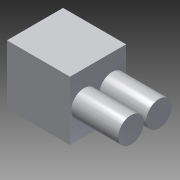
# Autodesk Inventor part: TE_2Pin_Male
Saved by Autodesk Inventor 2014 (Build 180170000, 170)
## iProperties
Created: 2015-04-19
Part Number: TE_2Pin_Male
Material: Generic
Document SubType Name: Modeling
Designer: Owner
Density: 1 g/cm^3
Appearance: White
Author: Owner
Autodesk Inventor part; units mm, degrees
ref_plane "YZ Plane" through (0, 0, 0) normal (1, 0, 0) x (0, 1, 0)
ref_plane "XZ Plane" through (0, 0, 0) normal (0, 1, 0) x (-1, 0, 0)
ref_plane "XY Plane" through (0, 0, 0) normal (0, 0, 1) x (1, 0, 0)
sketch "Sketch1" plane through (0, 0, 0) normal (0, 1, 0) x (-1, 0, 0)
  line L0 (-9.3023, 6.985) -> (6.3977, 6.985)
  line L1 (6.3977, 6.985) -> (6.3977, -6.985)
  line L2 (6.3977, -6.985) -> (-9.3023, -6.985)
  line L3 (-9.3023, -6.985) -> (-9.3023, 6.985)
  point P0 (0, 0)
  dimension "d0" = 13.97
  dimension "d1" = 15.7
  constraints: 8 end point, 2 parallel, 1 horizontal, 1 perpendicular
  measures "d0" distance of L0.end L1.end
  measures "d1" distance of L0.start L0.end
extrude "Extrusion1" add sketch "Sketch1" along normal blind 14.73
sketch "Sketch2" plane through (9.3023, 0, 6.985) normal (1, 0, 0) x (0, 0, -1)
  line L0 (13.97, 0) -> (13.97, 14.73) projected
  line L1 (0, 0) -> (0, 14.73) projected
  circle A0 centre (3.4925, 7.365) radius 3.175
  circle A1 centre (10.4775, 7.365) radius 3.175
  point P0 (6.985, 0)
  dimension "d4" = 3.4925
  dimension "d5" = 3.4925
  dimension "d6" = 6.35
  dimension "d7" = 6.35
  constraints: 2 centre point
  measures "d4" distance from line of L0 A1.centre
  measures "d5" distance from line of L1 A0.centre
  measures "d6" diameter of A0
  measures "d7" diameter of A1
extrude "Extrusion2" add sketch "Sketch2" along normal blind 11.68
body "Solid1"
